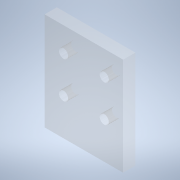
# Autodesk Inventor part: BaseC_9
Saved by Autodesk Inventor 2021 (Build 250183000, 183)
## iProperties
Created: 2023-10-23
Part Number: BaseC_9
Material: PMMA Plastic
Document SubType Name: Modeling
Designer: M
Density: 1.23759 g/cm^3
Appearance: Polycarbonate - Clear
Mass: 13.25 g
Surface Area: 49.4606 cm^2
Volume: 10.7063 cm^3
Author: M
Autodesk Inventor part; units mm, degrees
ref_plane "YZ Plane" through (0, 0, 0) normal (1, 0, 0) x (0, 1, 0)
ref_plane "XZ Plane" through (0, 0, 0) normal (0, 1, 0) x (-1, 0, 0)
ref_plane "XY Plane" through (0, 0, 0) normal (0, 0, 1) x (1, 0, 0)
sketch "Sketch1" plane through (0, 0, 0) normal (0, 0, 1) x (1, 0, 0)
  line L0 (0, 0) -> (38.5, 0)
  line L1 (0, 0) -> (0, 48)
  line L2 (0, 48) -> (38.5, 48)
  line L3 (38.5, 48) -> (38.5, 0)
  circle A0 centre (9.25, 18) radius 2.25
  line L4 (9.25, 18) -> (29.25, 18)
  circle A1 centre (29.25, 18) radius 2.25
  circle A2 centre (9.25, 36) radius 2.25
  line L5 (9.25, 36) -> (29.25, 36)
  circle A3 centre (29.25, 36) radius 2.25
  dimension "d0" = 48
  dimension "d3" = 18
  dimension "d4" = 4.5
  dimension "d5" = 4.5
  dimension "d6" = 20
  dimension "d7" = 38.5
  dimension "d8" = 9.25
  dimension "d9" = 4.5
  dimension "d10" = 4.5
  dimension "d11" = 20
  dimension "d12" = 12
  dimension "d13" = 9.25
  constraints: 12 end point, 4 centre point, 3 horizontal, 2 coincident, 2 perpendicular, 1 vertical
  measures "d0" distance of L0.start L1.end
  measures "d3" distance between parallel lines of L4 L0
  measures "d4" diameter of A0
  measures "d5" diameter of A1
  measures "d6" distance of L4.start L4.end
  measures "d7" distance of L1.end L2.end
  measures "d8" distance from line of L4.start L1
  measures "d9" diameter of A2
  measures "d10" diameter of A3
  measures "d11" distance of L5.start L5.end
  measures "d12" distance from line of L2 L5.start
  measures "d13" distance from line of L1 L5.start
extrude "Extrusion1" add sketch "Sketch1" along normal blind 6
equation "\"d5\" = d4"
equation "\"d8\" = -0.5 * d6 + 0.5 * d7"
equation "\"d10\" = d9"
equation "\"d13\" = -0.5 * d11 + 0.5 * d7"
body "Solid1"
